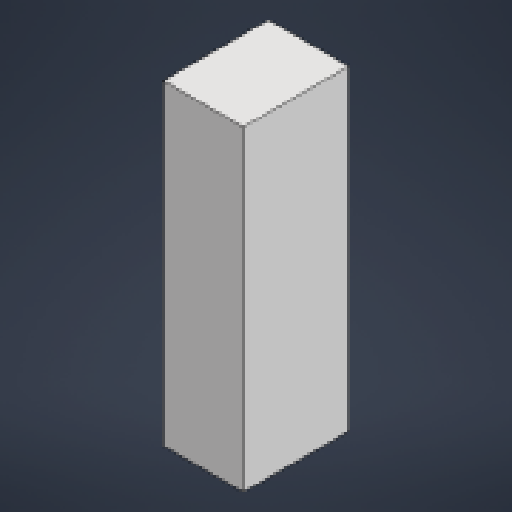
# Autodesk Inventor part: tattu
Saved by Autodesk Inventor 2023 (Build 270158000, 158)
## iProperties
Created: 2024-02-25
Part Number: tattu
Material: Generic
Document SubType Name: Modeling
Designer: Michał
Density: 1 g/cm^3
Appearance: Default
Author: Michał
Autodesk Inventor part; units mm, degrees
ref_plane "YZ Plane" through (0, 0, 0) normal (1, 0, 0) x (0, 1, 0)
ref_plane "XZ Plane" through (0, 0, 0) normal (0, 1, 0) x (-1, 0, 0)
ref_plane "XY Plane" through (0, 0, 0) normal (0, 0, 1) x (1, 0, 0)
sketch "Sketch1" plane through (0, 0, 0) normal (0, 0, 1) x (1, 0, 0)
  line L0 (-21.75, 23.25) -> (-5.75, 23.25)
  line L1 (-5.75, 23.25) -> (-5.75, -39.75)
  line L2 (-5.75, -39.75) -> (-21.75, -39.75)
  line L3 (-21.75, -39.75) -> (-21.75, 23.25)
  line L4 (-21.95, -42.75) -> (14.25, -42.75) construction
  line L5 (-21.95, -0.75) -> (-21.95, -42.75) construction
  point P0 (0, 0)
  dimension "d0" = 63
  dimension "d1" = 16
  dimension "d2" = 0.2
  dimension "d3" = 3
  constraints: 8 end point, 2 parallel, 1 horizontal, 1 perpendicular
  measures "d0" distance between parallel lines of L2 L0
  measures "d1" distance between parallel lines of L3 L1
  measures "d2" distance between parallel lines of L3 L5
  measures "d3" distance between parallel lines of L4 L2
extrude "Extrusion1" add sketch "Sketch1" along normal blind 21
body "Solid1"
